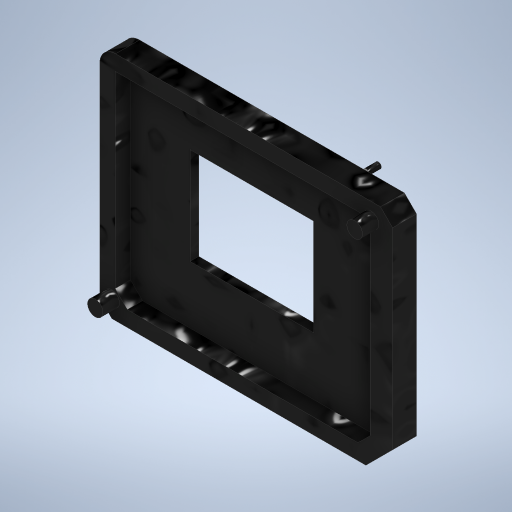
# Autodesk Inventor part: tray
Saved by Autodesk Inventor 2024 (Build 280153000, 153)
## iProperties
Created: 2024-09-23
Part Number: tray
Material: Generic
Document SubType Name: Modeling
Designer: PC
Density: 1 g/cm^3
Appearance: Default
Author: PC
Autodesk Inventor part; units mm, degrees
ref_plane "YZ Plane" through (0, 0, 0) normal (1, 0, 0) x (0, 1, 0)
ref_plane "XZ Plane" through (0, 0, 0) normal (0, 1, 0) x (-1, 0, 0)
ref_plane "XY Plane" through (0, 0, 0) normal (0, 0, 1) x (1, 0, 0)
sketch "Sketch1" plane through (0, 0, 0) normal (0, 0, 1) x (1, 0, 0)
  line L0 (2, 0) -> (43.86, 0)
  line L1 (48.26, 4.4) -> (48.26, 36.1)
  line L2 (46.26, 38.1) -> (2.6, 38.1)
  line L3 (0, 35.5) -> (0, 2)
  arc A0 (2.6, 38.1) -> (0, 35.5) centre (2.6, 35.5) ccw
  line L4 (2.54, 35.56) -> (42.54, 35.56)
  line L5 (44.54, 33.56) -> (44.54, 4.56)
  line L6 (42.54, 2.56) -> (4.54, 2.56)
  line L7 (2.54, 4.56) -> (2.54, 35.56)
  line L8 (43.86, 0) -> (48.26, 4.4)
  line L9 (44.54, 4.56) -> (42.54, 2.56)
  line L10 (4.54, 2.56) -> (2.54, 4.56)
  circle A1 centre (44.72, 35.43) radius 1.28
  circle A2 centre (1.97, 2.85) radius 1.27
  line L11 (2.54, 35.56) -> (44.54, 2.56) construction
  line L12 (44.54, 35.56) -> (2.54, 2.56) construction
  arc A3 (44.54, 33.56) -> (42.54, 35.56) centre (42.54, 33.56) ccw
  line L13 (48.26, 36.1) -> (46.26, 38.1)
  line L14 (2, 0) -> (0, 2)
  point P0 (0, 0)
  point P1 (48.26, 38.1)
  point P2 (48.26, 0)
  point P3 (0, 38.1)
  point P4 (4.2502, 2.8498)
  point P5 (2.916, 4.184)
  point P6 (43.4429, 35.3446)
  point P7 (44.4412, 34.1807)
  dimension "d0" = 38.1
  dimension "d1" = 48.26
  dimension "d2" = 2.6
  dimension "d3" = 33
  dimension "d4" = 42
  dimension "d5" = 2.54
  dimension "d6" = 2.54
  dimension "d7" = 4.4
  dimension "d8" = 4.4
  dimension "d9" = 2
  dimension "d10" = 2
  dimension "d11" = 2
  dimension "d12" = 2
  dimension "d13" = 44.72
  dimension "d14" = 2.56
  dimension "d15" = 2.67
  dimension "d16" = 2.54
  dimension "d27" = 2
  dimension "d28" = 2
  dimension "d29" = 2
  dimension "d30" = 1.97
  dimension "d31" = 2.85
  dimension "d32" = 2
  dimension "d33" = 2
  constraints: 30 end point, 14 point on line, 4 centre point, 4 parallel, 4 point on circle, 4 tangent, 2 horizontal, 2 perpendicular
  measures "d0" distance between parallel lines of L0 L2
  measures "d1" distance of point (48.26, 38.1) point (0, 38.1)
  measures "d2" radius of A0
  measures "d3" distance of L12.start L11.end
  measures "d4" distance of L4.start L12.start
  measures "d5" distance between parallel lines of L3 L7
  measures "d6" distance between parallel lines of L2 L4
  measures "d7" distance of L0.end point (48.26, 0)
  measures "d8" distance of L1.start point (48.26, 0)
  measures "d9" distance of L5.end L11.end
  measures "d10" distance of L6.start L11.end
  measures "d11" distance of L6.end L12.end
  measures "d12" distance of L7.start L12.end
  measures "d13" distance from line of L3 A1.centre
  measures "d14" diameter of A1
  measures "d15" distance from line of L2 A1.centre
  measures "d16" diameter of A2
  measures "d27" radius of A3
  measures "d28" distance of L1.end point (48.26, 38.1)
  measures "d29" distance of L2.start point (48.26, 38.1)
  measures "d30" distance from line of L3 A2.centre
  measures "d31" distance from line of L0 A2.centre
  measures "d32" distance of L0.start point (0, 0)
  measures "d33" distance of L3.end point (0, 0)
extrude "Extrusion1" add sketch "Sketch1" along normal blind 1.43 contours L14 L3 A0 L2 L13 L1 L8 L0 | L4 A3 A1 L5 L9 L6 L10 L7 | A3 A1 | A1 A3 | A2
extrude "Extrusion2" add sketch "Sketch1" along normal blind 3.95
extrude "Extrusion3" add sketch "Sketch1" along normal blind 4 contours A3 A1 | A1 A3 | A2
extrude "Extrusion4" add sketch "Sketch1" along normal blind 6.66 contours A3 A1 | A1 A3 | A2
sketch "Sketch2" plane through (0, 0, 1.43) normal (0, 0, 1) x (1, 0, 0)
  line L0 (12.36, 28.032) -> (32.72, 28.032)
  line L1 (32.72, 28.032) -> (32.72, 12.088)
  line L2 (32.72, 12.088) -> (12.36, 12.088)
  line L3 (12.36, 12.088) -> (12.36, 28.032)
  line L4 (2.54, 35.56) -> (42.54, 35.56) projected
  line L5 (2.54, 4.56) -> (2.54, 35.56) projected
  point P0 (0, 0)
  point P1 (22.54, 28.032)
  point P2 (22.54, 35.56)
  point P3 (2.54, 20.06)
  point P4 (12.36, 20.06)
  dimension "d34" = 25.86
  dimension "d35" = 20.36
  constraints: 8 end point, 4 midpoint, 2 parallel, 1 horizontal, 1 horizontal alignment, 1 perpendicular, 1 vertical alignment
  measures "d34" distance of L0.start L1.end
  measures "d35" distance of L1.end L2.end
extrude "Extrusion5" cut sketch "Sketch2" against normal blind 4
sketch "Sketch3" plane through (0, 0, 0) normal (0, 0, -1) x (-1, 0, 0)
  circle A0 centre (-39.96, 37.888) radius 0.4997
  circle A1 centre (-5.36, 2.788) radius 0.73
  line L0 (-2, 0) -> (-43.86, 0) projected
  line L1 (0, 35.5) -> (0, 2) projected
  line L2 (-46.26, 38.1) -> (-2.6, 38.1) projected
  line L3 (-12.36, 12.088) -> (-12.36, 28.032) projected
  point P0 (0, 0)
  dimension "d40" = 1.46
  dimension "d45" = 34.6
  dimension "d46" = 35.1
  dimension "d47" = 7
  dimension "d48" = 9.3
  constraints: 2 centre point
  measures "d40" diameter of A1
  measures "d45" horizontal distance of A1.centre A0.centre
  measures "d46" vertical distance of A0.centre A1.centre
  measures "d47" distance from line of A1.centre L3
  measures "d48" vertical distance of A1.centre L3.start
extrude "Extrusion6" add sketch "Sketch3" along normal blind 2
equation "\"d8\" = d7"
equation "\"d10\" = d9"
equation "\"d12\" = d11"
equation "\"d29\" = d28"
equation "\"d33\" = d32"
body "Solid1"
